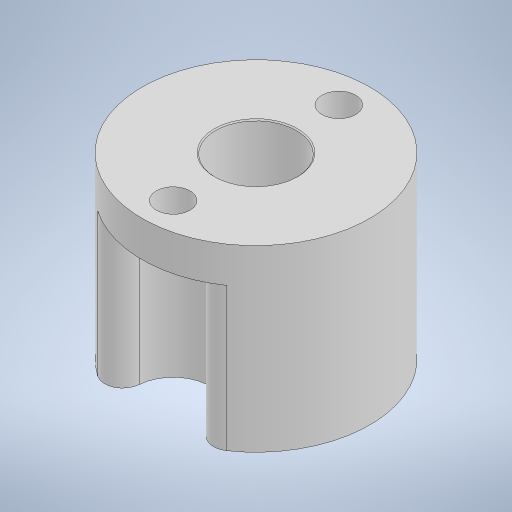
# Autodesk Inventor part: Core
Saved by Autodesk Inventor 2023.4 (Build 274418000, 418)
## iProperties
Created: 2024-05-29
Part Number: Core
Material: Generic
Document SubType Name: Modeling
Designer: Nathan Cai
Density: 1 g/cm^3
Appearance: Default
Author: Nathan Cai
Autodesk Inventor part; units mm, degrees
ref_plane "XZ Plane" through (0, 0, 0) normal (0, 1, 0) x (-1, 0, 0)
sketch "Sketch1" plane through (0, 0, 0) normal (0, 1, 0) x (-1, 0, 0)
  circle A0 centre (0, 0) radius 3.6
  circle A1 centre (0, 0) radius 10.1
  line L0 (0, 0) -> (10.1, 0) construction
  line L1 (0, 10.1) -> (0, 0) construction
  arc A2 (0, 4.6) -> (0, 10.1) centre (0, 7.35) ccw
  arc A3 (0, 4.6) -> (3.2527, 3.2527) centre (0, 0) ccw
  line L2 (0, -3.6) -> (0, -10.1) construction
  arc A4 (0, 4.1) -> (2.8991, 2.8991) centre (0, 0) ccw
  arc A5 (0, 4.1) -> (2.0201, 9.8959) centre (0, 7.35) ccw
  line L3 (7.1418, 7.1418) -> (0, 0) construction
  line L4 (3.2527, 3.2527) -> (2.8991, 2.8991)
  circle A6 centre (0, 7.35) radius 3.25
  point P0 (-9.3612, -3.7919)
  point P1 (-2.0201, 9.8959)
  dimension "d0" = 7.2
  dimension "d22" = 5.5
  dimension "d23" = 1
  dimension "d24" = 0.5
  constraints: 14 point on circle, 10 end point, 5 centre point, 5 point on line, 3 coincident, 3 tangent, 2 vertical, 1 collinear, 1 horizontal, 1 vertical alignment, 7 other
  measures "d22" diameter of A2
  measures "d24" radial gap between concentric circles of A3 A4
extrude "Extrusion1" add sketch "Sketch1" along normal blind 15.875 contours A1 A6 A3 L4 A4 A5 | A6 A4 L4 A3
fillet "Fillet3" radius 1.5875 2 edges at (2.0201, 7.9375, 9.8959) (-2.0201, 7.9375, 9.8959)
sketch "Sketch5" plane through (0, 15.875, 0) normal (0, 1, 0) x (1, 0, 0)
  arc A0 (5.7257, -8.3203) -> (-5.7257, -8.3203) centre (0, 0) ccw projected
  circle A1 centre (0, 0) radius 10.1
  arc A2 (3.2421, -7.1233) -> (-3.2421, -7.1233) centre (0, -7.35) ccw projected
  circle A3 centre (0, -7.35) radius 1.5
  circle A4 centre (0, 0) radius 3.6 projected
  dimension "d26" = 3
  constraints: 2 coincident, 1 centre point, 3 other
  measures "d26" diameter of A3
extrude "Extrusion5" add sketch "Sketch5" against normal blind 3.175
sketch "Sketch6" plane through (0, 15.875, 0) normal (0, 1, 0) x (1, 0, 0)
  circle A0 centre (0, -7.35) radius 1.5 projected
  circle A1 centre (0, 0) radius 7.35 construction
  circle A2 centre (0, 7.35) radius 1.5
  line L0 (0, 0) -> (0, 7.35) construction
  dimension "d32" = 3
  constraints: 2 centre point, 2 end point, 2 point on circle, 1 coincident, 1 vertical
  measures "d32" diameter of A2
extrude "Extrusion6" cut sketch "Sketch6" against normal blind 6.35 contours A2
chamfer "Chamfer2" distance 0.1 angle 45 2 edges at (3.6, 15.875, 0) (3.6, 0, 0)
sketch "Sketch2" plane through (0, 0, 0) normal (-0.7071068, 0, 0.7071068) x (0, -1, 0)
  line L0 (0, 10.1) -> (-15.875, 10.1) projected
  line L1 (-7.9375, 10.1) -> (-7.9375, -10.1) construction
  line L2 (0, -10.1) -> (-15.875, -10.1) projected
  circle A0 centre (-7.9375, 0) radius 1
  point P0 (0, 0)
  dimension "d8" = 2
  constraints: 3 midpoint, 2 end point, 1 centre point
  measures "d8" diameter of A0
sketch "Sketch3" plane through (-8.9803, 0, 8.9803) normal (-0.7071068, 0, 0.7071068) x (0, -1, 0)
  line L0 (0, 10.1) -> (-15.875, 10.1) projected
  line L1 (-7.9375, 10.1) -> (-7.9375, -10.1) construction
  line L2 (0, -10.1) -> (-15.875, -10.1) projected
  circle A0 centre (-7.9375, 0) radius 2
  point P0 (0, 0)
  dimension "d12" = 4
  constraints: 3 midpoint, 2 end point, 1 centre point
  measures "d12" diameter of A0
sketch "Sketch4" plane through (0, 15.875, 0) normal (0, 1, 0) x (1, 0, 0)
  line L0 (-5.85, 0) -> (-5.342, 0) projected
  circle A0 centre (0, 0) radius 5.342
  circle A1 centre (0, 0) radius 3.6 projected
  line L1 (0, 0) -> (6.0492, 0) construction
  arc A2 (0, -10.1) -> (-2.0201, -9.8959) centre (0, 0) ccw projected
  circle A3 centre (0, 0) radius 6.85
  line L2 (-9.8153, -2.3813) -> (9.8153, -2.3813)
  line L3 (9.8153, -2.3813) -> (9.8153, 2.3813) construction
  line L4 (9.8153, 2.3813) -> (-9.8153, 2.3812)
  line L5 (-9.8153, 2.3812) -> (-9.8153, -2.3813) construction
  line L6 (-9.8153, -2.3813) -> (9.8153, 2.3813) construction
  line L7 (9.8153, -2.3813) -> (-9.8153, 2.3812) construction
  line L8 (0, 0) -> (9.8153, 0) construction
  point P0 (0, 6.85)
  point P1 (-10.1, 0)
  point P2 (6.7726, -1.0269)
  point P3 (-4.7819, -2.3813)
  point P4 (4.7819, -2.3813)
  point P5 (-9.8153, -2.3813)
  point P6 (4.7819, 2.3813)
  point P7 (-4.7819, 2.3812)
  point P8 (-9.8153, 2.3812)
  point P9 (9.8153, -2.3813)
  point P10 (-8.6242, 5.2567)
  point P11 (-9.8153, 2.3812)
  point P12 (6.4228, 2.3813)
  point P13 (-6.4228, 2.3812)
  dimension "d20" = 4.7625
  dimension "d21" = 0
  constraints: 16 end point, 3 midpoint, 2 coincident, 2 parallel, 1 horizontal, 1 perpendicular, 8 other
  measures "d20" distance between parallel lines of L2 L4
  measures "d21" distance between parallel lines of L1 L8
body "Solid1"
